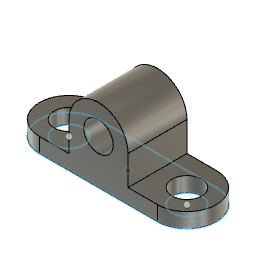
A4 v0 (Autodesk Fusion 360 design; units mm, degrees)
Autodesk Fusion 360 part; units mm, degrees
sketch "base" plane through (0, 0, 0) normal (0, 0, 1) x (1, 0, 0)
  line L0 (40, 20) -> (-40, 20)
  line L1 (-40, -20) -> (40, -20)
  circle A0 centre (-40, 0) radius 10
  circle A1 centre (40, 0) radius 10
  arc A2 (-40, 20) -> (-40, -20) centre (-40, 0) ccw
  arc A3 (40, -20) -> (40, 20) centre (40, 0) ccw
  dimension "d1" = 80
  dimension "d2" = 40
  dimension "d7" = 40
  dimension "d8" = 40
  dimension "d9" = 20
  dimension "d10" = 20
  constraint horizontal L0
  constraint parallel L0 L1
  constraint concentric A0 A2
  constraint concentric A1 A3
  measures "d1" distance of L1.start L1.end
  measures "d2" distance of L0.end L1.start
  measures "d7" diameter of A3
  measures "d8" diameter of A2
  measures "d9" diameter of A0
  measures "d10" diameter of A1
extrude "Extrude1" add sketch "base" along normal blind 10 contours L0 L1 A2 A3 | A0 | A1
extrude "Extrude2" cut 1 faces at (13.3333, -6.6667, 10) along direction (0, 0, -1) blind 10
extrude "Extrude3" add sketch "base" along normal blind 10
sketch "Sketch2" plane through (0, 0, 0) normal (0, 1, 0) x (1, 0, 0)
  line L0 (-20, 0) -> (20, 0)
  line L1 (20, 0) -> (20, -30)
  line L2 (-20, -30) -> (-20, 0)
  line L3 (-40, 0) -> (-40, -10)
  circle A0 centre (0, -30) radius 10
  arc A1 (-20, -30) -> (20, -30) centre (0, -30) ccw
  dimension "d15" = 40
  dimension "d18" = 30
  dimension "d19" = 20
  dimension "d20" = 40
  dimension "d21" = 20
  constraint horizontal L0
  constraint vertical L1
  constraint vertical L2
  constraint concentric A0 A1
  measures "d15" distance of L0.start L0.end
  measures "d18" distance of L0.start L2.start
  measures "d19" distance of L2 L3
  measures "d20" diameter of A1
  measures "d21" diameter of A0
extrude "Extrude4" add sketch "Sketch2" along normal mid plane 40
